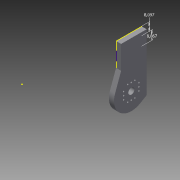
# Autodesk Inventor part: cadera
Saved by Autodesk Inventor 2015 (Build 190159000, 159)
## iProperties
Created: 2015-08-01
Part Number: cadera
Material: Genérico
Document SubType Name: Modeling
Designer: Roberto
Density: 1 g/cm^3
Appearance: Valor por defecto
Author: Roberto
Autodesk Inventor part; units mm, degrees
ref_plane "YZ Plane" through (0, 0, 0) normal (1, 0, 0) x (0, 1, 0)
ref_plane "XZ Plane" through (0, 0, 0) normal (0, 1, 0) x (-1, 0, 0)
ref_plane "XY Plane" through (0, 0, 0) normal (0, 0, 1) x (1, 0, 0)
ref_plane "Plano de trabajo1" through (129.4922, 102.1402, -54.3752) normal (1, 0, 0) x (0, 1, 0)
sketch "Boceto1" plane through (129.4922, 102.1402, -54.3752) normal (1, 0, 0) x (0, 1, 0)
  circle A0 centre (-7.5, 0) radius 0.75 projected
  circle A1 centre (3.5, 7.5) radius 0.75 projected
  circle A2 centre (-3.5, 7.5) radius 0.75 projected
  circle A3 centre (7.5, 0) radius 0.75 projected
  circle A4 centre (-3.5, -7.5) radius 0.75 projected
  circle A5 centre (0, -7.5) radius 0.75 projected
  circle A6 centre (3.5, -7.5) radius 0.75 projected
  circle A7 centre (7.5, 3.5) radius 0.75 projected
  circle A8 centre (7.5, -3.5) radius 0.75 projected
  circle A9 centre (0, 7.5) radius 0.75 projected
  circle A10 centre (-7.5, -3.5) radius 0.75 projected
  circle A11 centre (-7.5, 3.5) radius 0.75 projected
  circle A12 centre (0, 0) radius 3 projected
  circle A13 centre (0, 0) radius 10.5 projected
  arc A14 (-15.9748, 5.8143) -> (8.5, -14.7224) centre (0, 0) ccw
  line L0 (-15.9748, 5.8143) -> (-10, 22.2299)
  line L1 (-10, 22.2299) -> (-10, 45)
  line L2 (-10, 45) -> (15, 45)
  line L3 (15, 45) -> (15, -10.9697)
  line L4 (15, -10.9697) -> (8.5, -14.7224)
  point P0 (-102.1402, 54.3752)
  dimension "d0" = 17
  dimension "d1" = 45
  dimension "d2" = 10
  dimension "d3" = 25
  dimension "d4" = 160
  dimension "d5" = 60
  constraints: 10 end point, 3 point on circle, 2 perpendicular, 2 tangent, 1 centre point, 1 coincident, 1 vertical
  measures "d0" radius of A14
  measures "d1" distance from line of A12.centre L2
  measures "d2" distance from line of A12.centre L1
  measures "d3" distance of L1.end L2.end
  measures "d4" angle of L1 L0
  measures "d5" angle of L4 L3
extrude "Extrusión1" add sketch "Boceto1" along normal blind 5 contours A13 | L0 L1 L2 L3 L4 A14
sketch "Boceto2" plane through (129.4922, 102.1402, -54.3752) normal (-1, 0, 0) x (0, 0, 1)
  line L0 (35, -10) -> (28, -10)
  line L1 (28, -10) -> (28, 15)
  line L2 (28, 15) -> (35, 15)
  line L3 (35, 15) -> (35, -10)
  line L4 (45, -10) -> (22.2299, -10) projected
  line L5 (-10.9697, 15) -> (45, 15) projected
  line L6 (45, 15) -> (45, -10) projected
  point P0 (54.3752, -102.1402)
  dimension "d8" = 10
  dimension "d9" = 7
  constraints: 8 end point, 2 collinear, 2 parallel, 1 horizontal, 1 perpendicular
  measures "d8" distance between parallel lines of L6 L3
  measures "d9" distance of L1.end L2.end
extrude "Extrusión2" add sketch "Boceto2" along normal blind 55.5 contours L0 L1 L2 L3
sketch "Boceto4" plane through (73.9922, 102.1402, -54.3752) normal (-1, 0, 0) x (0, 0, 1)
  line L0 (35, 15) -> (28, 15) projected
  line L1 (35, 15) -> (45, 15) projected
  line L2 (45, 15) -> (45, -10) projected
  line L3 (45, -10) -> (35, -10) projected
  line L4 (28, -10) -> (35, -10) projected
  line L5 (-10.9697, 15) -> (28, 15) projected
  circle A0 centre (0, 0) radius 1.8 projected
  line L6 (-10.9697, 15) -> (45, 15) projected
  arc A1 (-7.8826, -1.3657) -> (6.6543, -4.4407) centre (0, 0) ccw
  arc A2 (1.0303, 15) -> (-7.8826, -1.3657) centre (6.8973, 1.195) ccw
  line L7 (28, -10) -> (25, -10)
  arc A3 (25, -10) -> (6.6543, -4.4407) centre (14.9848, -10) ccw
  point P0 (54.3752, -102.1402)
  dimension "d20" = 8
  dimension "d21" = 12
  dimension "d23" = 15
  dimension "d24" = 20
  constraints: 6 point on circle, 3 centre point, 2 end point, 2 tangent, 1 collinear, 1 concentric, 1 line through centre, 1 point on line
  measures "d20" radius of A1
  measures "d21" distance of L5.start A2.start
  measures "d23" radius of A2
  measures "d24" distance of L2.end L7.end
extrude "Extrusión4" add sketch "Boceto4" along normal blind 4
